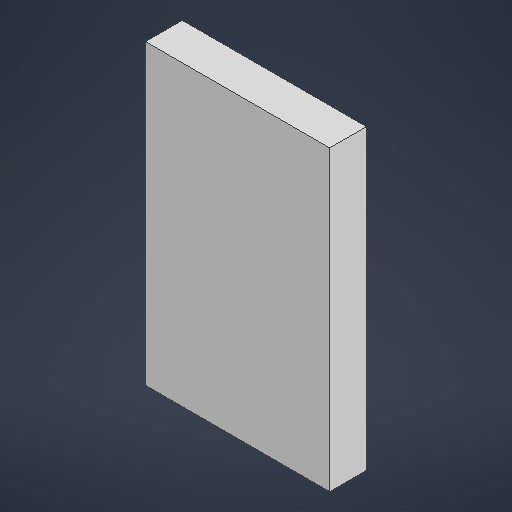
# Autodesk Inventor part: Part1
Saved by Autodesk Inventor 2026 (Build 300175000, 175)
## iProperties
Created: 2026-03-02
Part Number: Part1
Material: Generic
Document SubType Name: Modeling
Designer: shahd
Density: 1 g/cm^3
Appearance: Default
Author: shahd
Autodesk Inventor part; units mm, degrees
ref_plane "YZ Plane" through (0, 0, 0) normal (1, 0, 0) x (0, 1, 0)
ref_plane "XZ Plane" through (0, 0, 0) normal (0, 1, 0) x (-1, 0, 0)
ref_plane "XY Plane" through (0, 0, 0) normal (0, 0, 1) x (1, 0, 0)
sketch "Sketch1" plane through (0, 0, 0) normal (0, 0, 1) x (1, 0, 0)
  line L0 (0, 0) -> (10.0065, 0)
  line L1 (10.0065, 0) -> (10.0065, 16.1735)
  line L2 (10.0065, 16.1735) -> (0, 16.1735)
  line L3 (0, 16.1735) -> (0, 0)
  constraints: 8 end point, 2 parallel, 1 horizontal, 1 perpendicular
extrude "Extrusion1" add sketch "Sketch1" along normal blind 2
body "Solid1"
